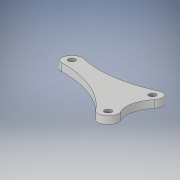
# Autodesk Inventor part: 連接2
Saved by Autodesk Inventor 2017 (Build 210142000, 142)
## iProperties
Part Number: 連接2
Material: 一般
Document SubType Name: Modeling
Designer: User
Density: 1 g/cm^3
Appearance: 預設
Author: User
Autodesk Inventor part; units mm, degrees
ref_plane "YZ Plane" through (0, 0, 0) normal (1, 0, 0) x (0, 1, 0)
ref_plane "XZ Plane" through (0, 0, 0) normal (0, 1, 0) x (-1, 0, 0)
ref_plane "XY Plane" through (0, 0, 0) normal (0, 0, 1) x (1, 0, 0)
sketch "草圖1" plane through (0, 0, 0) normal (0, 1, 0) x (-1, 0, 0)
  circle A0 centre (0, 0) radius 1.5
  line L0 (0, 0) -> (-40, 0)
  circle A1 centre (-40, 0) radius 1.5
  line L1 (-40, 0) -> (-41.7431, 19.9239)
  circle A2 centre (-41.7431, 19.9239) radius 1.5
  circle A3 centre (0, 0) radius 4
  circle A4 centre (-40, 0) radius 4
  circle A5 centre (-41.7431, 19.9239) radius 4
  arc A6 (-43.4405, 2.0403) -> (-44.7771, 17.3172) centre (-54.7513, 8.7476) ccw
  arc A7 (-1.3167, -3.7771) -> (-38.6833, -3.7771) centre (-20, -57.374) ccw
  arc A8 (-38.9519, 22.789) -> (0.4722, 3.972) centre (8.4988, 71.4966) ccw
  dimension "d0" = 3
  dimension "d1" = 40
  dimension "d2" = 3
  dimension "d3" = 95
  dimension "d4" = 20
  dimension "d5" = 3
  dimension "d6" = 8
  dimension "d7" = 8
  dimension "d8" = 8
  dimension "d9" = 13.15
  dimension "d10" = 56.76
  dimension "d11" = 68
  constraints: 12 point on circle, 9 centre point, 6 coincident, 6 tangent, 4 end point, 1 horizontal
  measures "d0" diameter of A0
  measures "d1" distance of L0.start L0.end
  measures "d2" diameter of A1
  measures "d3" angle of L1 L0
  measures "d4" distance of L1.start L1.end
  measures "d5" diameter of A2
  measures "d6" diameter of A3
  measures "d7" diameter of A4
  measures "d8" diameter of A5
  measures "d9" radius of A6
  measures "d10" radius of A7
  measures "d11" radius of A8
extrude "擠出1" add sketch "草圖1" along normal mid plane 3 contours A3 | A3 A7 A4 L0 | L0 A4 L1 A5 A8 A3 | A4 L1 A1 L0 | L0 A1 L1 A4 | A4 A6 A5 L1 | A5
